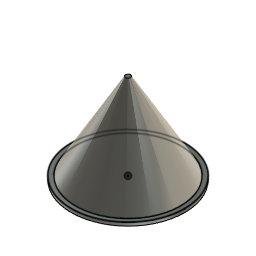
V60FilterConeHolder (Autodesk Fusion 360 design; units mm, degrees)
Autodesk Fusion 360 part; units mm, degrees
sketch "Sketch1" plane through (0, 0, 0) normal (0, 0, 1) x (1, 0, 0)
  circle A0 centre (0, 0) radius 60
  circle A1 centre (0, 0) radius 65
  dimension "diameter" = 120
  dimension "d6" = 130
  constraint coincident A0.centre A1.centre
  measures "diameter" diameter of A0
  measures "d6" diameter of A1
extrude "Extrude1" add sketch "Sketch1" along normal blind 98.923 draft -30 contours A0
extrude "Extrude2" add sketch "Sketch1" against normal blind 4 contours A0 | A1
equation "diameter = FilterDiameter + 10 mm"
equation "d2 = diameter / 2 / tan(30 deg) - 5 mm"
equation "d6 = diameter + 10 mm"
equation "FilterDiameter = 110 mm" comment "No1=100, No2=110, No3=???"
